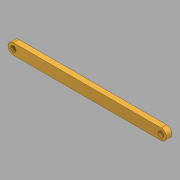
# Autodesk Inventor part: Link
Saved by Autodesk Inventor 2020 (Build 240168000, 168)
## iProperties
Created: 2019-11-25
Part Number: Link
Material: Latón, amarillo claro
Document SubType Name: Modeling
Designer: Gerardo Naranjo
Density: 8.47 g/cm^3
Appearance: Latón - Satinado
Engineer: Gerardo Naranjo
Author: Gerardo Naranjo
Title: Link
Autodesk Inventor part; units mm, degrees
ref_plane "YZ Plane" through (0, 0, 0) normal (1, 0, 0) x (0, 1, 0)
ref_plane "XZ Plane" through (0, 0, 0) normal (0, 1, 0) x (-1, 0, 0)
ref_plane "XY Plane" through (0, 0, 0) normal (0, 0, 1) x (1, 0, 0)
sketch "Boceto1" plane through (0, 0, 0) normal (0, 0, 1) x (1, 0, 0)
  line L0 (0, 0) -> (-42.8625, 0)
  line L1 (-42.8625, 3.175) -> (0, 3.175)
  arc A0 (-42.8625, 3.175) -> (-42.8625, 0) centre (-42.8625, 1.5875) ccw
  arc A1 (0, 0) -> (0, 3.175) centre (0, 1.5875) ccw
  circle A2 centre (-42.8625, 1.5875) radius 0.7938
  circle A3 centre (0, 1.5875) radius 0.7937
  dimension "d0" = 42.8625
  dimension "d5" = 3.175
  dimension "d6" = 3.175
  dimension "d7" = 1.5875
  dimension "d8" = 1.5875
  constraints: 4 centre point, 4 end point, 4 point on circle, 3 tangent, 2 coincident, 1 horizontal, 1 parallel
  measures "d0" distance of L1.start L1.end
  measures "d5" diameter of A0
  measures "d6" diameter of A1
  measures "d7" diameter of A2
  measures "d8" diameter of A3
extrude "Extrusión1" add sketch "Boceto1" along normal blind 1.5875
